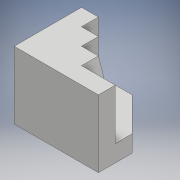
# Autodesk Inventor part: 15
Saved by Autodesk Inventor 2017 (Build 210142000, 142)
## iProperties
Part Number: 15
Material: 一般
Document SubType Name: Modeling
Designer: Brian
Density: 1 g/cm^3
Appearance: 預設
Author: Brian
Autodesk Inventor part; units mm, degrees
ref_plane "YZ Plane" through (0, 0, 0) normal (1, 0, 0) x (0, 1, 0)
ref_plane "XZ Plane" through (0, 0, 0) normal (0, 1, 0) x (-1, 0, 0)
ref_plane "XY Plane" through (0, 0, 0) normal (0, 0, 1) x (1, 0, 0)
sketch "草圖1" plane through (0, 0, 0) normal (0, 1, 0) x (-1, 0, 0)
  line L0 (0, 0) -> (-50, 0)
  line L1 (-50, 0) -> (-50, -40)
  line L2 (-50, -40) -> (0, -40)
  line L3 (0, -40) -> (0, 0)
  dimension "d0" = 50
  dimension "d1" = 40
  constraints: 8 end point, 2 parallel, 1 horizontal, 1 perpendicular
  measures "d0" distance of L1.end L2.end
  measures "d1" distance of L2.end L0.start
extrude "擠出1" add sketch "草圖1" along normal blind 10
sketch "草圖2" plane through (0, 10, 0) normal (0, 1, 0) x (1, 0, 0)
  line L0 (50, 40) -> (0, 40) projected
  line L1 (-0.0002, 40) -> (50, 40)
  line L2 (50, 40) -> (50, 30)
  line L3 (50, 0) -> (50, 40) projected
  line L4 (50, 30) -> (40, 30)
  line L5 (40, 30) -> (30, 0)
  line L6 (0, 0) -> (50, 0) projected
  line L7 (0, 0) -> (30, 0)
  line L8 (0, 0) -> (0, 40)
  dimension "d4" = 10
  dimension "d5" = 10
  dimension "d6" = 10
  constraints: 12 end point, 3 point on line, 2 horizontal, 1 collinear, 1 perpendicular
  measures "d4" distance of L2.end L4.end
  measures "d5" horizontal distance of L4.end L5.end
  measures "d6" distance between parallel lines of L0 L4
extrude "擠出2" add sketch "草圖2" along normal blind 10 contours L2 L4 L5 L6 L8 L0
sketch "草圖3" plane through (0, 20, 0) normal (0, 1, 0) x (1, 0, 0)
  line L0 (50, 40) -> (0, 40) projected
  line L1 (0, 40) -> (10, 40)
  line L2 (10, 40) -> (10, 0)
  line L3 (10, 0) -> (0, 0)
  line L4 (0, 0) -> (0, 40)
  line L5 (50, 40) -> (10, 40)
  line L6 (10, 40) -> (10, 30)
  line L7 (10, 30) -> (50, 30)
  line L8 (50, 30) -> (50, 40)
  point P0 (0, 0)
  dimension "d9" = 10
  dimension "d10" = 40
  dimension "d11" = 10
  constraints: 16 end point, 4 parallel, 2 horizontal, 2 perpendicular, 1 point on line
  measures "d9" distance between parallel lines of L4 L2
  measures "d10" distance of L3.end L0.end
  measures "d11" distance between parallel lines of L0 L7
extrude "擠出3" add sketch "草圖3" along normal blind 20
sketch "草圖4" plane through (40, 10, -30) normal (0, 0, 1) x (1, 0, 0)
  line L0 (0, 10) -> (-30, 10) projected
  line L1 (-30, 10) -> (-20, 10)
  line L2 (-20, 10) -> (-20, 20)
  line L3 (-20, 20) -> (-30, 20)
  line L4 (-30, 20) -> (-30, 10)
  point P0 (-40, -10)
  dimension "d14" = 10
  dimension "d15" = 10
  constraints: 8 end point, 2 parallel, 1 horizontal, 1 perpendicular
  measures "d14" distance of L2.end L3.end
  measures "d15" distance of L1.end L2.end
extrude "擠出4" add sketch "草圖4" along normal up to surface (30 mm away)
chamfer "倒角1" distance 20 angle 45 1 edges at (50, 40, -35)
